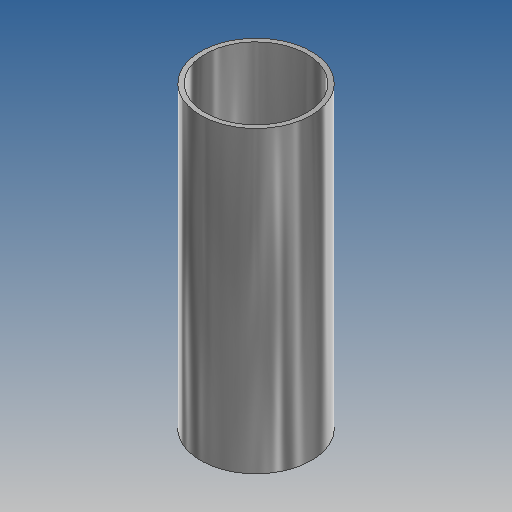
# Autodesk Inventor part: P024
Saved by Autodesk Inventor 2021.4 (Build 254397000, 397)
## iProperties
Company: HES-SO
Created: 2022-06-11
Part Number: P024
Material: Aluminium
Document SubType Name: Modeling
Designer: HER & ZAE
Density: 2.7 g/cm^3
Appearance: Aluminum - Dark
Author: HER & ZAE
Title: Entretoise Roulements
Autodesk Inventor part; units mm, degrees
ref_plane "YZ Plane" through (0, 0, 0) normal (1, 0, 0) x (0, 1, 0)
ref_plane "XZ Plane" through (0, 0, 0) normal (0, 1, 0) x (-1, 0, 0)
ref_plane "XY Plane" through (0, 0, 0) normal (0, 0, 1) x (1, 0, 0)
sketch "Sketch2" plane through (0, 0, 0) normal (0, 0, 1) x (1, 0, 0)
  circle A0 centre (0, 0) radius 8.5
  circle A1 centre (0, 0) radius 9.25
  dimension "d0" = 17
  dimension "d1" = 18.5
  constraints: 2 centre point, 2 coincident
  measures "d0" diameter of A0
  measures "d1" diameter of A1
extrude "Extrusion1" add sketch "Sketch2" along normal blind 50
body "Solid1"
